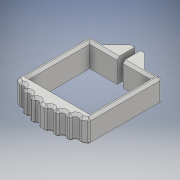
# Autodesk Inventor part: Fitness_rygmaskine_Fod
Saved by Autodesk Inventor 2018 (Build 220112000, 112)
## iProperties
Created: 2018-12-05
Part Number: Fitness_rygmaskine_Fod
Material: Generic
Document SubType Name: Modeling
Designer: JARVIS
Density: 1 g/cm^3
Appearance: Default
Author: JARVIS
Autodesk Inventor part; units mm, degrees
ref_plane "YZ Plane" through (0, 0, 0) normal (1, 0, 0) x (0, 1, 0)
ref_plane "XZ Plane" through (0, 0, 0) normal (0, 1, 0) x (-1, 0, 0)
ref_plane "XY Plane" through (0, 0, 0) normal (0, 0, 1) x (1, 0, 0)
sketch "Sketch2" plane through (0, 0, 0) normal (0, 0, 1) x (1, 0, 0)
  line L0 (31, 31) -> (31, -31)
  line L1 (-31, -31) -> (-31, 31)
  arc A0 (-31, -31) -> (31, -31) centre (0, 15) ccw
  line L2 (-16, 31) -> (-6, 41)
  line L3 (-6, 41) -> (6, 41)
  line L4 (6, 41) -> (16, 31)
  line L5 (-31, 31) -> (-16, 31)
  line L6 (16, 31) -> (31, 31)
  line L7 (-26, 26) -> (26, 26)
  line L8 (26, 26) -> (26, -26)
  line L9 (26, -26) -> (-26, -26)
  line L10 (-26, -26) -> (-26, 26)
  point P0 (0, 0)
  point P1 (0, 41)
  point P2 (0, 26)
  point P3 (26, 0)
  dimension "d2" = 52
  dimension "d3" = 135
  dimension "d4" = 135
  dimension "d5" = 15
  dimension "d6" = 5
  dimension "d7" = 5
  dimension "d9" = 12
  dimension "d10" = 5
  dimension "d11" = 10
  constraints: 22 end point, 4 horizontal, 3 equal length, 3 midpoint, 3 parallel, 3 perpendicular, 3 vertical alignment, 2 point on circle, 1 centre point, 1 horizontal alignment
  measures "d2" distance of L7.start L7.end
  measures "d3" angle of L2 L5
  measures "d4" angle of L6 L4
  measures "d5" distance of point (0, 0) A0.centre
  measures "d6" distance between parallel lines of L10 L1
  measures "d7" distance between parallel lines of L7 L6
  measures "d9" distance of L2.end L3.end
  measures "d10" distance from line of L0.end L9
  measures "d11" distance from line of L4.end L3
extrude "Extrusion1" add sketch "Sketch2" along normal mid plane 20
sketch "Sketch4" plane through (-6, 41, 10) normal (0, 1, 0) x (1, 0, 0)
  line L0 (0, 20) -> (0, 0) projected
  line L1 (12, 0) -> (0, 0) projected
  line L2 (12, 20) -> (12, 0) projected
  line L3 (0, 20) -> (12, 20) projected
  line L4 (-20, 0) -> (32, 0) projected
  line L5 (32, 20) -> (-20, 20) projected
  line L6 (3.5, 0) -> (8.5, 0)
  line L7 (8.5, 0) -> (8.5, 20)
  line L8 (8.5, 20) -> (3.5, 20)
  line L9 (3.5, 20) -> (3.5, 0)
  point P0 (6, 10)
  point P1 (6, 20)
  dimension "d14" = 5
  constraints: 8 end point, 2 parallel, 2 point on line, 1 horizontal, 1 midpoint, 1 perpendicular, 1 vertical alignment
  measures "d14" distance between parallel lines of L9 L7
extrude "Extrusion2" cut sketch "Sketch4" against normal blind 20 contours L3 L7 L1 L9
sketch "Sketch6" plane through (0, 0, 0) normal (0, 0, 1) x (1, 0, 0)
  line L0 (-6, 41) -> (-16, 31) projected
  line L1 (-16, 31) -> (-6, 31)
  line L2 (-6, 31) -> (-6, 41)
  line L3 (-6, 41) -> (-16, 31)
  point P0 (0, 0)
  constraints: 6 end point, 1 collinear, 1 horizontal, 1 perpendicular
extrude "Extrusion3" cut sketch "Sketch6" along normal mid plane 12
mirror "Mirror1" about plane through (0, 0, 0) normal (1, 0, 0) of "Extrusion3"
sketch "Sketch7" plane through (-6, 31, -6) normal (-1, 0, 0) x (0, 0, 1)
  arc A0 (4.2764, 3.5537) -> (4.2764, 6.4463) centre (6, 5) ccw
  line L0 (4.2764, 3.5537) -> (3.0628, 5)
  line L1 (3.0628, 5) -> (4.2764, 6.4463)
  line L2 (0, 10) -> (0, 0) projected
  line L3 (0, 10) -> (12, 10) projected
  point P0 (6, -31)
  point P1 (0, 5)
  point P2 (6, 10)
  dimension "d19" = 4.5
  dimension "d20" = 100
  constraints: 4 end point, 2 horizontal alignment, 2 midpoint, 2 point on circle, 2 tangent, 1 centre point, 1 vertical alignment
  measures "d19" diameter of A0
  measures "d20" angle of L1 L0
extrude "Extrusion4" cut sketch "Sketch7" against normal through all
sketch "Sketch8" plane through (0, 0, 10) normal (0, 0, 1) x (1, 0, 0)
  arc A0 (-31, -31) -> (31, -31) centre (0, 15) ccw projected
  circle A1 centre (-23.1532, -35.4076) radius 2.5
  circle A2 centre (-14.6969, -38.4883) radius 2.5
  circle A3 centre (-5.8537, -40.161) radius 2.5
  point P0 (0, 0)
  dimension "d23" = 5
  dimension "d24" = 9
  dimension "d25" = 9
  dimension "d26" = 9
  constraints: 3 centre point, 3 point on circle, 2 equal radius
  measures "d23" diameter of A1
  measures "d24" distance of A0.start A1.centre
  measures "d25" distance of A1.centre A2.centre
  measures "d26" distance of A2.centre A3.centre
extrude "Extrusion5" cut sketch "Sketch8" against normal through all
mirror "Mirror2" about plane through (0, 0, 0) normal (1, 0, 0) of "Extrusion5"
fillet "Fillet1" radius 2 16 edges at (-25.4009, -34.3132, 0) (-20.8584, -36.3997, 0) (-17.092, -37.7718, 0) (-12.2719, -39.0962, 0) (-8.3331, -39.8412, 0) (-3.3623, -40.3687, 0) (3.3623, -40.3687, 0) (8.3331, -39.8412, 0) (12.2719, -39.0962, 0) (17.092, -37.7718, 0) (20.8584, -36.3997, 0) (25.4009, -34.3132, 0) (-31, -31, 0) (31, -31, 0) (-31, 31, 0) (31, 31, 0)
chamfer "Chamfer1" distance 2 angle 45 5 edges at (0, -26, 10) (-26, 0, 10) (26, 0, 10) (14.25, 26, 10) (-14.25, 26, 10)
chamfer "Chamfer2" distance 2 angle 45 66 edges at (17.4828, -37.3173, 10) (14.0345, -36.0777, 10) (11.7037, -38.9052, 10) (10.3092, -39.5043, 10) (8.7923, -39.4559, 10) (5.5898, -37.6749, 10) (2.8325, -40.0883, 10) (0, -40.4707, 10) (-2.8325, -40.0883, 10) (-5.5898, -37.6749, 10) (-8.7923, -39.4559, 10) (-10.3092, -39.5043, 10) (-11.7037, -38.9052, 10) (-14.0345, -36.0777, 10) (-17.4828, -37.3173, 10) (-18.9876, -37.1198, 10) (-20.2668, -36.303, 10) (-22.1097, -33.1358, 10) (-25.7131, -33.8015, 10) (-28.4682, -32.6084, 10) (-30.7563, -30.8802, 10) (-31, -0.4617, 10) (-30.4142, 30.4142, 10) (-22.5, 31, 10) (18.9876, -37.1198, 10) (20.2668, -36.303, 10) (22.1097, -33.1358, 10) (25.7131, -33.8015, 10) (28.4682, -32.6084, 10) (30.7563, -30.8802, 10) (31, -0.4617, 10) (30.4142, 30.4142, 10) (22.5, 31, 10) (20.2668, -36.303, -10) (22.1097, -33.1358, -10) (25.7131, -33.8015, -10) (28.4682, -32.6084, -10) (30.7563, -30.8802, -10) (31, -0.4617, -10) (30.4142, 30.4142, -10) (22.5, 31, -10) (18.9876, -37.1198, -10) (17.4828, -37.3173, -10) (14.0345, -36.0777, -10) (11.7037, -38.9052, -10) (10.3092, -39.5043, -10) (8.7923, -39.4559, -10) (5.5898, -37.6749, -10) (2.8325, -40.0883, -10) (0, -40.4707, -10) (-2.8325, -40.0883, -10) (-5.5898, -37.6749, -10) (-8.7923, -39.4559, -10) (-10.3092, -39.5043, -10) (-11.7037, -38.9052, -10) (-14.0345, -36.0777, -10) (-17.4828, -37.3173, -10) (-18.9876, -37.1198, -10) (-20.2668, -36.303, -10) (-22.1097, -33.1358, -10) (-25.7131, -33.8015, -10) (-28.4682, -32.6084, -10) (-30.7563, -30.8802, -10) (-31, -0.4617, -10) (-30.4142, 30.4142, -10) (-22.5, 31, -10)
equation "\"d4\" = d3"
equation "\"d7\" = d6"
equation "\"d10\" = d6"
equation "\"d25\" = d24"
equation "\"d26\" = d24"
body "Solid1"
